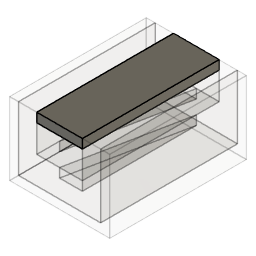
V4.2 (Autodesk Fusion 360 design; units mm, degrees)
part number: 2026-06-11-15-33-25-034
part number: 2026-06-11-15-39-48-904
part number: 2026-06-11-15-42-00-713
part number: 2026-06-11-15-44-55-864
part number: 2026-06-11-15-46-27-976
part number: 2026-06-11-15-51-44-010
part number: 2026-06-11-15-55-50-120
Autodesk Fusion 360 part; units mm, degrees
sketch "Esquisse1" plane through (0, 0, 0) normal (1, 0, 0) x (0, 1, 0)
sketch "Esquisse2" plane through (0, 0, 0) normal (0, 0, 1) x (1, 0, 0)
  line L0 (0, 0) -> (22, 0)
  line L1 (22, 0) -> (22, 30)
  line L2 (22, 30) -> (0, 30)
  line L3 (0, 30) -> (0, 0)
  dimension "d10" = 22
  dimension "d11" = 30
  constraint horizontal L0
  constraint vertical L1
  constraint horizontal L2
  constraint vertical L3
  constraint coincident L0.start L3.end
  measures "d10" distance of L0.start L0.end
  measures "d11" distance of L0.start L2.end
sketch "Esquisse3" plane through (0, 0, 0) normal (0, 0, 1) x (1, 0, 0)
  line L0 (0, 0) -> (2, 0)
  line L1 (2, 0) -> (2, 30)
  line L2 (2, 30) -> (0, 30)
  line L3 (0, 30) -> (0, 0)
  dimension "d12" = 2
  dimension "d13" = 30
  constraint horizontal L0
  constraint vertical L1
  constraint horizontal L2
  constraint vertical L3
  constraint coincident L0.start L3.end
  measures "d12" distance of L0.start L0.end
  measures "d13" distance of L0.start L2.end
sketch "Esquisse4" plane through (0, 0, 0) normal (0, 0, 1) x (1, 0, 0)
  line L0 (22, 0) -> (20, 0)
  line L1 (20, 0) -> (20, 30)
  line L2 (20, 30) -> (22, 30)
  line L3 (22, 30) -> (22, 0)
  dimension "d14" = 2
  dimension "d15" = 30
  constraint horizontal L0
  constraint vertical L1
  constraint horizontal L2
  constraint vertical L3
  measures "d14" distance of L0.start L0.end
  measures "d15" distance of L0.start L2.end
sketch "Esquisse1 (2)" plane through (0, 0, 0) normal (0, 0, 1) x (1, 0, 0) in component "shield"
extrude "Extrusion1" add sketch "Esquisse3" along normal blind 16 makes body 1 in component "shield"
extrude "Extrusion2" add sketch "Esquisse4" along normal blind 16 separate body makes body 2 in component "shield"
extrude "Extrusion3" add sketch "Esquisse2" along normal blind 2 bodies 1 2 in component "shield"
sketch "Esquisse2 (2)" plane through (0, 0, 2) normal (0, 0, 1) x (-1, 0, 0) in component "shield"
  line L0 (-2, -30) -> (-2, 0)
  line L1 (-2, 0) -> (-20, 0)
  line L2 (-20, 0) -> (-20, -30)
  line L3 (-20, -30) -> (-2, -30)
  line L4 (-2, -30) -> (-6, -30)
  line L5 (-6, -30) -> (-6, 0)
  line L6 (-6, 0) -> (-2, 0)
  line L7 (-2, 0) -> (-2, -30)
  line L8 (-20, -30) -> (-16, -30)
  line L9 (-16, -30) -> (-16, 0)
  line L10 (-16, 0) -> (-20, 0)
  line L11 (-20, 0) -> (-20, -30)
  dimension "d22" = 4
  dimension "d23" = 30
  dimension "d24" = 4
  dimension "d25" = 30
  constraint horizontal L4
  constraint vertical L5
  constraint horizontal L6
  constraint vertical L7
  constraint coincident L0.start L3.end
  constraint horizontal L8
  constraint vertical L9
  constraint horizontal L10
  constraint vertical L11
  constraint coincident L2.end L3.start
  measures "d22" distance of L0.start L4.end
  measures "d23" distance of L0.start L0.end
  measures "d24" distance of L2.end L8.end
  measures "d25" distance of L2.end L1.end
extrude "Extrusion1'" add sketch "Esquisse2 (2)" along normal blind 14 separate body contours L0 L1 L3 L4 L5 L6 L7 | L1 L2 L3 L8 L9 L10 L11 makes body 3 at (6, 20, 6.6667) makes body 4 at (20, 10, 6.6667) in component "Support"
sketch "Esquisse1 (3)" plane through (0, 0, 2) normal (0, 0, 1) x (-1, 0, 0) in component "Support"
  line L0 (-2, -30) -> (-2, 0)
  line L1 (-2, 0) -> (-20, 0)
  line L2 (-20, 0) -> (-20, -30)
  line L3 (-20, -30) -> (-2, -30)
  line L4 (-16, -30) -> (-6, -30)
  line L5 (-6, -30) -> (-6, 0)
  line L6 (-6, 0) -> (-16, 0)
  line L7 (-16, 0) -> (-16, -30)
  dimension "d28" = 10
  dimension "d29" = 30
  constraint horizontal L4
  constraint vertical L5
  constraint horizontal L6
  constraint vertical L7
  constraint coincident L3 L4.start
  measures "d28" distance of L4.start L4.end
  measures "d29" distance of L4.start L6.end
extrude "Extrusion2'" add sketch "Esquisse1 (3)" along normal blind 4 contours L1 L3 L4 L5 L6 L7 bodies 3 4 in component "Support"
sketch "Esquisse1 (4)" plane through (0, 0, 6) normal (0, 0, 1) x (-1, 0, 0) in component "trianglee_1"
  line L0 (-16, 0) -> (-16, -30)
  line L1 (-16, -30) -> (-6, -30)
  line L2 (-6, -30) -> (-6, 0)
  line L3 (-6, 0) -> (-16, 0)
  spline S0 degree 5 poles (-11, 0) (-11.2, -1) (-11.6, -3) (-12.2, -6) (-13, -10) (-14, -15) (-14.8, -19) (-15.4, -22) (-15.8, -24) (-16, -25) knots 0 0 0 0 0 0 0.2 0.4 0.6 0.8 1 1 1 1 1 1
  dimension "d32" = 5
  dimension "d33" = 5
  constraint coincident L3 S0.start
  constraint coincident L0 S0.end
  measures "d32" distance of L2.end S0.start
  measures "d33" distance of L0.end S0.end
extrude "Extrusion1''" add sketch "Esquisse1 (4)" along normal blind 2 separate body contours L0 L3 S0 makes body 5 in component "trianglee_1"
sketch "Esquisse1 (5)" plane through (0, 0, 6) normal (0, 0, 1) x (-1, 0, 0) in component "triangle_2"
  line L0 (-16, 0) -> (-16, -30)
  line L1 (-16, -30) -> (-6, -30)
  line L2 (-6, -30) -> (-6, 0)
  line L3 (-6, 0) -> (-16, 0)
  spline S0 degree 5 poles (-6, -5) (-6.2, -6) (-6.6, -8) (-7.2, -11) (-8, -15) (-9, -20) (-9.8, -24) (-10.4, -27) (-10.8, -29) (-11, -30) knots 0 0 0 0 0 0 0.2 0.4 0.6 0.8 1 1 1 1 1 1
  dimension "d36" = 5
  dimension "d37" = 5
  constraint coincident L2 S0.start
  constraint coincident L1 S0.end
  measures "d36" distance of L0.end S0.end
  measures "d37" distance of L2.end S0.start
extrude "Extrusion1'''" add sketch "Esquisse1 (5)" along normal blind 2 separate body contours L1 L2 S0 makes body 6 in component "triangle_2"
extrude "Extrusion3'" add 1 faces at (12.6667, 20, 6) along direction (0, 0, 1) blind 2 on bodies 3 bodies 3 in component "Support"
copy_body "CopierCollerCorps1" bodies 5 makes body 7 in component "Support"
copy_body "CopierCollerCorps2" bodies 6 makes body 8 in component "Support"
combine "Combiner1" operation cut target body 3 tool bodies 7 8 in component "Support"
sketch "Esquisse1 (6)" plane through (0, 0, 8) normal (0, 0, 1) x (-1, 0, 0) in component "Mousse"
  line L0 (-11, -30) -> (-6, -5)
  line L1 (-6, -5) -> (-6, 0)
  line L2 (-6, 0) -> (-11, 0)
  line L3 (-11, 0) -> (-16, -25)
  line L4 (-16, -25) -> (-16, -30)
  line L5 (-16, -30) -> (-11, -30)
  line L6 (-6, -30) -> (-16, -30)
  line L7 (-16, -30) -> (-16, 0)
  line L8 (-16, 0) -> (-6, 0)
  line L9 (-6, 0) -> (-6, -30)
  constraint horizontal L6
  constraint vertical L7
  constraint horizontal L8
  constraint vertical L9
extrude "Extrusion1''''" add sketch "Esquisse1 (6)" along normal blind 6 separate body makes body 9 in component "Mousse"
extrude "Extrusion1'''''" add 1 faces at (12.6667, 10, 14) along direction (0, 0, 1) blind 2 separate body on bodies 9 makes body 10 in component "plateau"
component "shield" placed x (1, 0, 0) y (0, 1, 0) z (0, 0, 1) at (0, 0, 0)
component "Support" placed x (1, 0, 0) y (0, 1, 0) z (0, 0, 1) at (0, 0, 0)
component "trianglee_1" placed x (1, 0, 0) y (0, 1, 0) z (0, 0, 1) at (0, 0, 0)
component "triangle_2" placed x (1, 0, 0) y (0, 1, 0) z (0, 0, 1) at (0, 0, 0)
component "Mousse" placed x (1, 0, 0) y (0, 1, 0) z (0, 0, 1) at (0, 0, 0)
component "plateau" placed x (1, 0, 0) y (0, 1, 0) z (0, 0, 1) at (0, 0, 0)
equation "épaisseur_mousse = 6 mm"
equation "distance_bord = 4 mm"
equation "epaisseur = 2 mm"
equation "distance_plaques = 5 mm"
equation "Longueur = 30 mm"
equation "hauteur = distance_bord + 3 * epaisseur + épaisseur_mousse"
equation "largeur_base_triangle = 5 mm"
equation "largeur = 2 * distance_bord + 2 * epaisseur + distance_plaques + largeur_base_triangle"
equation "d10 = largeur"
equation "d11 = Longueur"
equation "d12 = epaisseur"
equation "d13 = Longueur"
equation "d14 = epaisseur"
equation "d15 = Longueur"
equation "d16 = hauteur"
equation "d18 = hauteur"
equation "d20 = epaisseur"
equation "d22 = distance_bord"
equation "d23 = Longueur"
equation "d24 = distance_bord"
equation "d25 = Longueur"
equation "d26 = hauteur - epaisseur"
equation "d28 = distance_plaques + largeur_base_triangle"
equation "d29 = Longueur"
equation "d30 = distance_bord"
equation "d32 = distance_plaques"
equation "d33 = distance_plaques"
equation "d34 = epaisseur"
equation "d36 = distance_plaques"
equation "d37 = distance_plaques"
equation "d38 = epaisseur"
equation "d40 = epaisseur"
equation "d42 = épaisseur_mousse"
equation "d44 = epaisseur"
